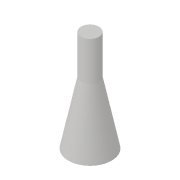
# Autodesk Inventor part: control stick
Saved by Autodesk Inventor 2018 (Build 220112000, 112)
## iProperties
Created: 2019-02-02
Part Number: control stick
Material: Generic
Document SubType Name: Modeling
Designer: ball
Density: 1 g/cm^3
Appearance: Default
Author: ball
Autodesk Inventor part; units mm, degrees
ref_plane "YZ Plane" through (0, 0, 0) normal (1, 0, 0) x (0, 1, 0)
ref_plane "XZ Plane" through (0, 0, 0) normal (0, 1, 0) x (-1, 0, 0)
ref_plane "XY Plane" through (0, 0, 0) normal (0, 0, 1) x (1, 0, 0)
sketch "Sketch1" plane through (0, 0, 0) normal (0, 0, 1) x (1, 0, 0)
  line L0 (0, 0) -> (4.2164, 0)
  line L1 (0, 0) -> (0, 12.1158)
  line L2 (0, 12.1158) -> (1.7399, 12.1158)
  line L3 (1.7399, 12.1158) -> (4.2164, 0)
  line L4 (0, 12.1158) -> (1.7399, 12.1158)
  line L5 (1.7399, 12.1158) -> (1.7399, 19.7358)
  line L6 (1.7399, 19.7358) -> (0, 19.7358)
  line L7 (0, 19.7358) -> (0, 12.1158)
  dimension "d0" = 4.2164
  dimension "d1" = 12.1158
  dimension "d2" = 1.7399
  dimension "d3" = 7.62
  dimension "d5" = 1.7399
  constraints: 16 end point, 3 horizontal, 2 parallel, 1 perpendicular, 1 vertical
  measures "d0" distance of L0.start L0.end
  measures "d1" distance of L0.start L1.end
  measures "d2" distance of L1.end L2.end
  measures "d3" distance of L5.end L4.end
  measures "d5" distance between parallel lines of L5 L7
revolve "Revolution1" add sketch "Sketch1" angle 360 about axis through (0, 0, 0) along (0, 1, 0)
body "Solid1"
